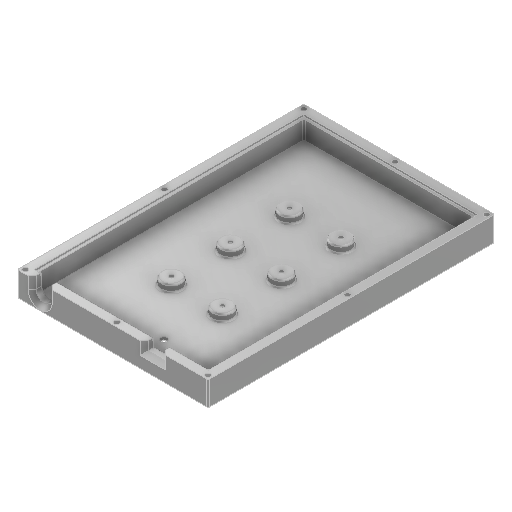
# Autodesk Inventor part: 3DP_PLA_Back_Cover
Saved by Autodesk Inventor 2026.1 (Build 301233000, 233)
## iProperties
Created: 2024-08-15
Part Number: 3DP_PLA_Back_Cover
Material: Generic
Document SubType Name: Modeling
Designer: User
Density: 1 g/cm^3
Appearance: Rubber - Black - Version 1.1
Author: User
Autodesk Inventor part; units mm, degrees
ref_plane "YZ Plane" through (0, 0, 0) normal (1, 0, 0) x (0, 1, 0)
ref_plane "XZ Plane" through (0, 0, 0) normal (0, 1, 0) x (-1, 0, 0)
ref_plane "XY Plane" through (0, 0, 0) normal (0, 0, 1) x (1, 0, 0)
sketch "Sketch1" plane through (0, 0, 0) normal (0, 1, 0) x (-1, 0, 0)
  line L0 (64.5, 100) -> (-64.5, 100)
  line L1 (-64.5, 100) -> (-64.5, -100)
  line L2 (-64.5, -100) -> (64.5, -100)
  line L3 (64.5, -100) -> (64.5, 100)
  line L4 (-65, 100.5) -> (65, 100.5)
  line L5 (65, 100.5) -> (65, -100.5)
  line L6 (65, -100.5) -> (-65, -100.5)
  line L7 (-65, -100.5) -> (-65, 100.5)
  line L8 (71, -106.5) -> (71, 106.5)
  line L9 (71, 106.5) -> (-71, 106.5)
  line L10 (-71, 106.5) -> (-71, -106.5)
  line L11 (-71, -106.5) -> (71, -106.5)
  line L12 (63, -98.5) -> (63, 98.5)
  line L13 (63, 98.5) -> (-63, 98.5)
  line L14 (-63, 98.5) -> (-63, -98.5)
  line L15 (-63, -98.5) -> (63, -98.5)
  line L16 (-64.7, 100.2) -> (64.7, 100.2)
  line L17 (64.7, 100.2) -> (64.7, -100.2)
  line L18 (64.7, -100.2) -> (-64.7, -100.2)
  line L19 (-64.7, -100.2) -> (-64.7, 100.2)
  point P0 (0, 0)
  dimension "d0" = 200
  dimension "d1" = 129
  dimension "d2" = 64.5
  dimension "d3" = 100
  dimension "d4" = 0.5
  dimension "d5" = 6
  dimension "d8" = 2
  dimension "d77" = 0.2
  constraints: 40 end point, 10 parallel, 5 perpendicular, 1 horizontal, 12 other
  measures "d0" distance of L2.end L0.start
  measures "d1" distance of L0.start L0.end
  measures "d2" distance from line of point (0, 0) L3
  measures "d3" distance from line of L0 point (0, 0)
  measures "d4" distance between parallel lines of L0 L4
  measures "d5" distance between parallel lines of L5 L8
  measures "d8" distance between parallel lines of L5 L12
  measures "d77" distance between parallel lines of L0 L16
extrude "Extrusion1" add sketch "Sketch1" against normal blind 15 contours L3 L2 L1 L0 | L4 L5 L6 L7 | L11 L10 L9 L8 | L16 L17 L18 L19
extrude "Extrusion2" cut sketch "Sketch1" against normal blind 1.6 contours L3 L2 L1 L0 | L16 L17 L18 L19
sketch "Sketch2" plane through (0, -15, 0) normal (0, -1, 0) x (1, 0, 0)
  line L0 (71, 106.5) -> (-71, 106.5) projected
  line L1 (-71, 106.5) -> (-71, -106.5) projected
  line L2 (-71, -106.5) -> (71, -106.5) projected
  line L3 (71, -106.5) -> (71, 106.5) projected
  line L4 (63, -98.5) -> (-63, -98.5) projected
  line L5 (-63, -98.5) -> (-63, 98.5) projected
  line L6 (-63, 98.5) -> (63, 98.5) projected
  line L7 (63, 98.5) -> (63, -98.5) projected
  point P0 (0, 0)
extrude "Extrusion3" add sketch "Sketch2" along normal blind 3 contours L3 L2 L1 L0 | L4 L5 L6 L7
sketch "Sketch4" plane through (-71, 0, 106.5) normal (0, 0, 1) x (1, 0, 0)
  line L0 (8, -15) -> (134, -15) projected
  line L1 (8, -1.6) -> (8, -15) projected
  line L2 (134, -1.6) -> (134, -15) projected
  circle A0 centre (17, -8.6) radius 6
  line L3 (96.85, -1.6) -> (104.35, -1.6)
  line L4 (104.35, -1.6) -> (104.35, -4.1)
  line L5 (104.35, -4.1) -> (96.85, -4.1)
  line L6 (96.85, -4.1) -> (96.85, -1.6)
  line L7 (106.85, -6.6) -> (106.85, 0.9)
  line L8 (106.85, 0.9) -> (94.35, 0.9)
  line L9 (94.35, 0.9) -> (94.35, -6.6)
  line L10 (94.35, -6.6) -> (106.85, -6.6)
  line L11 (11, -8.6) -> (11, 0)
  line L12 (142, 0) -> (0, 0) projected
  line L13 (23, -8.6) -> (23, 0)
  line L14 (135.7, -1.6) -> (6.3, -1.6) projected
  line L15 (6.3, 0) -> (6.3, -1.6) projected
  line L16 (135.7, 0) -> (135.7, -1.6) projected
  point P0 (71, 0)
  dimension "d13" = 9
  dimension "d15" = 12
  dimension "d16" = 29.65
  dimension "d17" = 7.5
  dimension "d19" = 2.5
  dimension "d78" = 8.6
  dimension "d79" = 4.1
  constraints: 20 end point, 5 parallel, 2 perpendicular, 2 point on circle, 2 point on line, 1 centre point, 1 horizontal, 1 vertical, 3 other
  measures "d13" distance from line of L1 A0.centre
  measures "d15" diameter of A0
  measures "d16" distance between parallel lines of L2 L4
  measures "d17" distance between parallel lines of L4 L6
  measures "d19" distance between parallel lines of L4 L7
  measures "d78" distance from line of L12 A0.centre
  measures "d79" distance between parallel lines of L12 L5
extrude "Extrusion4" cut sketch "Sketch4" against normal blind 10 contours L14 L13 A0 L11 | L11 L12 L13 L14 | L14 L3 L9 L12 L7 | L7 L10 L9 L14 L6 L5 L4 | A0 | L12 L9 L8 L7 | L4 L5 L6 L3
chamfer "Chamfer2" distance 3 angle 45 3 edges at (35.85, -3.3, 106.5) (29.6, -6.6, 106.5) (23.35, -3.3, 106.5)
chamfer "Chamfer3" distance 3 angle 45 3 edges at (-54, -14.6, 106.5) (-60, -4.3, 106.5) (-48, -4.3, 106.5)
sketch "Sketch5" plane through (0, 0, 0) normal (0, 1, 0) x (1, 0, 0)
  line L0 (-60, -103.5) -> (-63, -106.5) projected
  line L1 (-60, -103.5) -> (-60, -100.2) projected
  line L2 (35.85, -100.2) -> (35.85, -103.5) projected
  line L3 (38.85, -106.5) -> (35.85, -103.5) projected
  line L4 (38.85, -106.5) -> (71, -106.5) projected
  line L5 (71, -106.5) -> (71, 106.5) projected
  line L6 (71, 106.5) -> (-71, 106.5) projected
  line L7 (-71, 106.5) -> (-71, -106.5) projected
  line L8 (-71, -106.5) -> (-63, -106.5) projected
  line L9 (-45, -106.5) -> (-48, -103.5) projected
  line L10 (-45, -106.5) -> (20.35, -106.5) projected
  line L11 (23.35, -103.5) -> (20.35, -106.5) projected
  line L12 (23.35, -103.5) -> (23.35, -100.2) projected
  line L13 (-48, -100.2) -> (-48, -103.5) projected
  line L14 (23.35, -100.2) -> (-48, -100.2) projected
  line L15 (-60, -100.2) -> (-64.7, -100.2) projected
  line L16 (-64.7, -100.2) -> (-64.7, 100.2) projected
  line L17 (-64.7, 100.2) -> (64.7, 100.2) projected
  line L18 (64.7, 100.2) -> (64.7, -100.2) projected
  line L19 (64.7, -100.2) -> (35.85, -100.2) projected
  point P0 (0, 0)
  point P1 (68, 103.5)
  point P2 (68, 0)
  point P3 (68, -103.5)
  point P4 (-68, 103.5)
  point P5 (-68, 0)
  point P6 (-68, -103.5)
  point P7 (0, -103.5)
  point P8 (0, 103.5)
  dimension "d33" = 3
  dimension "d34" = 3
  dimension "d36" = 106.5
  dimension "d37" = 213
  dimension "d38" = 3
  dimension "d39" = 3
  dimension "d40" = 3
  dimension "d41" = 71
  dimension "d42" = 142
  constraints: 5 horizontal alignment, 3 vertical alignment
  measures "d33" distance from line of L5 point (68, 103.5)
  measures "d34" distance from line of L6 point (68, 103.5)
  measures "d36" distance from line of L4 point (68, 0)
  measures "d37" distance between parallel lines of L6 L4
  measures "d38" distance from line of L5 point (68, -103.5)
  measures "d39" distance from line of L4 point (68, -103.5)
  measures "d40" distance from line of L7 point (-68, 103.5)
  measures "d41" distance from line of L5 point (0, 103.5)
  measures "d42" distance between parallel lines of L7 L5
hole "Hole1" at (68, 0, -103.5) at (68, 0, 0) at (68, 0, 103.5) at (-68, 0, -103.5) at (-68, 0, 0) at (-68, 0, 103.5) at (0, 0, 103.5) at (0, 0, -103.5) direction (0, -1, 0) diameter 4 depth 6.5
sketch "Sketch6" plane through (0, -18, 0) normal (0, -1, 0) x (1, 0, 0)
  line L0 (-63, 98.5) -> (63, 98.5) projected
  line L1 (63, 98.5) -> (63, -98.5) projected
  line L2 (-63, -98.5) -> (-63, 98.5) projected
  line L3 (63, -98.5) -> (-63, -98.5) projected
  point P0 (0, 0)
  point P1 (13.5, 93)
  point P2 (13.5, 82)
  dimension "d50" = 49.5
  dimension "d51" = 5.5
  dimension "d52" = 11
  constraints: 1 vertical alignment
  measures "d50" distance from line of L1 point (13.5, 82)
  measures "d51" distance from line of L0 point (13.5, 93)
  measures "d52" distance of point (13.5, 93) point (13.5, 82)
hole "Hole2" at (13.5, -18, 93) at (13.5, -18, 82) direction (0, 1, 0) diameter 5 end through all
chamfer "Chamfer4" distance 1 angle 45 2 edges at (13.5, -18, 95.5) (13.5, -18, 84.5)
sketch "Sketch7" plane through (0, -18, 0) normal (0, -1, 0) x (1, 0, 0)
  line L0 (8.5616, 95.7266) -> (8.5616, 75.4371) construction
  line L1 (8.5616, 75.4371) -> (2.563, 75.4371) construction
  line L2 (2.563, 75.4371) -> (2.563, 95.7266) construction
  line L3 (2.563, 95.7266) -> (8.5616, 95.7266) construction
  line L4 (2.5616, 89.5613) -> (2.5616, 91.3944)
  line L5 (2.5616, 91.3944) -> (4.7642, 93.0621)
  line L6 (4.7642, 93.0621) -> (4.7642, 93.6067)
  line L7 (4.7642, 93.6067) -> (2.5616, 93.6067)
  line L8 (2.5616, 93.6067) -> (2.5616, 95.1043)
  line L9 (2.5616, 95.1043) -> (8.5616, 95.1043)
  line L10 (8.5616, 95.1043) -> (8.5616, 92.6926)
  spline S0 degree 2 poles (8.5616, 92.6926) (8.5616, 92.1918) (8.4352, 91.4527) (8.2407, 91.1367) knots 0 0 0 1 2 2 2
  spline S1 degree 2 poles (8.2407, 91.1367) (8.0365, 90.8158) (7.3996, 90.4365) (6.9133, 90.4365) knots 0 0 0 1 2 2 2
  spline S2 degree 2 poles (6.9133, 90.4365) (6.2278, 90.4365) (5.3672, 91.0589) (5.1143, 91.5791) knots 0 0 0 1 2 2 2
  line L11 (5.1143, 91.5791) -> (2.5616, 89.5613)
  spline S3 degree 2 poles (6.7237, 91.9827) (6.9522, 91.9827) (7.278, 92.1577) (7.3655, 92.3571) knots 0 0 0 1 2 2 2
  spline S4 degree 2 poles (7.3655, 92.3571) (7.4239, 92.4981) (7.4579, 92.8433) (7.4579, 93.101) knots 0 0 0 1 2 2 2
  line L12 (7.4579, 93.101) -> (7.4579, 93.6067)
  line L13 (7.4579, 93.6067) -> (5.8437, 93.6067)
  line L14 (5.8437, 93.6067) -> (5.8437, 93.174)
  spline S5 degree 2 poles (5.8437, 93.174) (5.8437, 92.8628) (5.9215, 92.4203) (6.043, 92.2696) knots 0 0 0 1 2 2 2
  spline S6 degree 2 poles (6.043, 92.2696) (6.1597, 92.1237) (6.4709, 91.9827) (6.7237, 91.9827) knots 0 0 0 1 2 2 2
  spline S7 degree 2 poles (6.6702, 79.6667) (6.2521, 79.6667) (5.4936, 79.9341) (5.2407, 80.1821) knots 0 0 0 1 2 2 2
  spline S8 degree 2 poles (5.2407, 80.1821) (5.0803, 80.3328) (4.8177, 80.7023) (4.7253, 80.9211) knots 0 0 0 1 2 2 2
  spline S9 degree 2 poles (4.7253, 80.9211) (4.633, 81.1448) (4.526, 81.665) (4.526, 81.986) knots 0 0 0 1 2 2 2
  line L15 (4.526, 81.986) -> (4.526, 82.7736)
  line L16 (4.526, 82.7736) -> (2.5616, 82.7736)
  line L17 (2.5616, 82.7736) -> (2.5616, 84.2809)
  line L18 (2.5616, 84.2809) -> (8.5616, 84.2809)
  line L19 (8.5616, 84.2809) -> (8.5616, 81.9519)
  spline S10 degree 2 poles (8.5616, 81.9519) (8.5616, 81.4365) (8.372, 80.6829) (8.1678, 80.3766) knots 0 0 0 1 2 2 2
  spline S11 degree 2 poles (8.1678, 80.3766) (7.9393, 80.0362) (7.1905, 79.6667) (6.6702, 79.6667) knots 0 0 0 1 2 2 2
  spline S12 degree 2 poles (6.6313, 81.2129) (6.889, 81.2129) (7.2537, 81.456) (7.3218, 81.6213) knots 0 0 0 1 2 2 2
  spline S13 degree 2 poles (7.3218, 81.6213) (7.4142, 81.8352) (7.4433, 82.2242) (7.4433, 82.5597) knots 0 0 0 1 2 2 2
  line L20 (7.4433, 82.5597) -> (7.4433, 82.7736)
  line L21 (7.4433, 82.7736) -> (5.6443, 82.7736)
  line L22 (5.6443, 82.7736) -> (5.6443, 82.6667)
  spline S14 degree 2 poles (5.6443, 82.6667) (5.6443, 82.4576) (5.654, 82.0783) (5.6783, 81.9373) knots 0 0 0 1 2 2 2
  spline S15 degree 2 poles (5.6783, 81.9373) (5.6978, 81.8158) (5.8145, 81.5483) (5.8874, 81.4754) knots 0 0 0 1 2 2 2
  spline S16 degree 2 poles (5.8874, 81.4754) (6.0333, 81.3198) (6.3591, 81.2129) (6.6313, 81.2129) knots 0 0 0 1 2 2 2
  point P0 (0, 0)
  constraints: 2 other
extrude "Extrusion5" cut sketch "Sketch7" against normal blind 0.5
fillet "Fillet1" radius 1 14 edges at (63, -8.3, -98.5) (63, -8.3, 98.5) (-63, -8.3, 98.5) (-63, -8.3, -98.5) (-71, -9, -106.5) (71, -9, -106.5) (-71, -9, 106.5) (71, -9, 106.5) (23.35, -4.1, 98.5) (35.85, -4.1, 98.5) (29.6, -6.6, 98.5) (-48, -5.1, 98.5) (-60, -5.1, 98.5) (-54, -14.6, 98.5)
sketch "Sketch8" plane through (0, -18, 0) normal (0, -1, 0) x (1, 0, 0)
  line L0 (19, 44) -> (-19, 44)
  line L1 (-19, 44) -> (-19, -44)
  line L2 (-19, -44) -> (19, -44)
  line L3 (19, -44) -> (19, 44)
  point P0 (0, 0)
  point P1 (-19, 0)
  point P2 (19, 0)
  dimension "d66" = 38
  dimension "d67" = 88
  dimension "d68" = 44
  dimension "d69" = 19
  constraints: 8 end point, 4 coincident, 2 midpoint, 2 parallel, 1 horizontal, 1 perpendicular
  measures "d66" distance of L2.end L1.end
  measures "d67" distance of L1.end L0.end
  measures "d68" distance from line of L0 point (0, 0)
  measures "d69" distance from line of L3 point (0, 0)
hole "Hole3" at (19, -18, 44) at (-19, -18, 44) at (-19, -18, 0) at (-19, -18, -44) at (19, -18, -44) at (19, -18, 0) direction (0, 1, 0) diameter 4 depth 6.5
hole "Hole4" at (-68, 0, 103.5) at (-68, 0, 0) at (0, 0, 103.5) at (68, 0, 103.5) at (68, 0, 0) at (68, 0, -103.5) at (0, 0, -103.5) at (-68, 0, -103.5) direction (0, -1, 0) diameter 3.5 depth 15
sketch "Sketch9" plane through (0, -15, 0) normal (0, 1, 0) x (1, 0, 0)
  circle A0 centre (19, 0) radius 2 projected
  circle A1 centre (19, 44) radius 2 projected
  circle A2 centre (-19, 44) radius 2 projected
  circle A3 centre (-19, 0) radius 2 projected
  circle A4 centre (-19, -44) radius 2 projected
  circle A5 centre (19, -44) radius 2 projected
  circle A6 centre (13.5, -82) radius 2.5 projected
  circle A7 centre (13.5, -93) radius 2.5 projected
  arc A8 (-62, 98.5) -> (-63, 97.5) centre (-62, 97.5) ccw projected
  line L0 (-63, 97.5) -> (-63, -97.5) projected
  arc A9 (-63, -97.5) -> (-62, -98.5) centre (-62, -97.5) ccw projected
  line L1 (-62, -98.5) -> (-56.8355, -98.5) projected
  line L2 (-51.1645, -98.5) -> (62, -98.5) projected
  arc A10 (62, -98.5) -> (63, -97.5) centre (62, -97.5) ccw projected
  line L3 (63, -97.5) -> (63, 97.5) projected
  arc A11 (63, 97.5) -> (62, 98.5) centre (62, 97.5) ccw projected
  line L4 (62, 98.5) -> (-62, 98.5) projected
  circle A12 centre (19, 44) radius 7.5
  circle A13 centre (19, 0) radius 7.5
  circle A14 centre (19, -44) radius 7.5
  circle A15 centre (-19, 44) radius 7.5
  circle A16 centre (-19, 0) radius 7.5
  circle A17 centre (-19, -44) radius 7.5
  point P0 (0, 0)
  dimension "d87" = 15
  dimension "d88" = 15
  dimension "d89" = 15
  dimension "d90" = 15
  dimension "d91" = 15
  dimension "d92" = 15
  constraints: 6 centre point, 6 coincident, 1 horizontal alignment
  measures "d87" diameter of A12
  measures "d88" diameter of A13
  measures "d89" diameter of A14
  measures "d90" diameter of A15
  measures "d91" diameter of A16
  measures "d92" diameter of A17
extrude "Extrusion6" add sketch "Sketch9" along normal blind 3.5 contours A12 | A13 | A14 | A15 | A16 | A17
sketch "Sketch10" plane through (-19, -11.5, 0) normal (0, 1, 0) x (1, 0, 0)
  circle A0 centre (38, 44) radius 7.5 projected
  circle A1 centre (38, 44) radius 2 projected
  circle A2 centre (38, 0) radius 7.5 projected
  circle A3 centre (38, 0) radius 2 projected
  circle A4 centre (38, -44) radius 7.5 projected
  circle A5 centre (38, -44) radius 2 projected
  circle A6 centre (0, -44) radius 7.5 projected
  circle A7 centre (0, -44) radius 2 projected
  circle A8 centre (0, 0) radius 7.5 projected
  circle A9 centre (0, 0) radius 2 projected
  circle A10 centre (0, 44) radius 7.5 projected
  circle A11 centre (0, 44) radius 2 projected
  circle A12 centre (38, 44) radius 1.75
  circle A13 centre (38, 0) radius 1.75
  circle A14 centre (38, -44) radius 1.75
  circle A15 centre (0, 44) radius 1.75
  circle A16 centre (0, 0) radius 1.75
  circle A17 centre (0, -44) radius 1.75
  point P0 (19, 0)
  dimension "d95" = 3.5
  dimension "d96" = 3.5
  dimension "d97" = 3.5
  dimension "d98" = 3.5
  dimension "d99" = 3.5
  dimension "d100" = 3.5
  constraints: 6 centre point, 6 coincident
  measures "d95" diameter of A12
  measures "d96" diameter of A13
  measures "d97" diameter of A14
  measures "d98" diameter of A15
  measures "d99" diameter of A16
  measures "d100" diameter of A17
extrude "Extrusion7" add sketch "Sketch10" along normal blind 2 contours A0 | A1 | A2 | A3 | A4 | A5 | A6 | A7 | A8 | A9 | A10 | A11
chamfer "Chamfer5" distance 0.25 angle 45 6 edges at (17.25, -11.5, 44) (-20.75, -11.5, 44) (-20.75, -11.5, 0) (17.25, -11.5, 0) (17.25, -11.5, -44) (-20.75, -11.5, -44)
chamfer "Chamfer6" distance 1 angle 45 12 edges at (11.5, -15, -44) (-26.5, -15, -44) (-26.5, -15, 0) (11.5, -15, 0) (11.5, -15, 44) (-26.5, -15, 44) (-26.5, -9.5, 44) (11.5, -9.5, 44) (11.5, -9.5, 0) (-26.5, -9.5, 0) (-26.5, -9.5, -44) (11.5, -9.5, -44)
equation "\"d2\" = 0.5 * d1"
equation "\"d3\" = 0.5 * d0"
equation "\"d33\" = 0.5 * d32"
equation "\"d34\" = d33"
equation "\"d41\" = 0.5 * d42"
equation "\"d68\" = 0.5 * d67"
equation "\"d69\" = 0.5 * d66"
equation "\"d32\" = 6"
body "Solid1"
